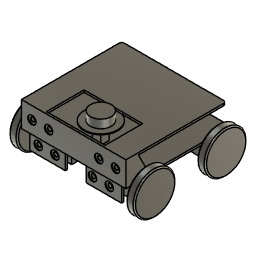
warehouse_robo v1 (Autodesk Fusion 360 design; units mm, degrees)
Autodesk Fusion 360 part; units mm, degrees
sketch "Sketch1" plane through (0, 0, 0) normal (0, 0, 1) x (1, 0, 0)
  line L0 (125, 125) -> (-125, 125)
  line L1 (-125, 125) -> (-125, -125)
  line L2 (-125, -125) -> (125, -125)
  line L3 (125, -125) -> (125, 125)
  line L4 (125, 125) -> (-125, -125) construction
  line L5 (-125, 125) -> (125, -125) construction
  dimension "d1" = 250
  dimension "d2" = 250
  constraint horizontal L0
  constraint perpendicular L0 L1
  constraint parallel L0 L2
  constraint parallel L1 L3
  constraint coincident L4 origin
  constraint coincident L5 origin
  measures "d1" distance of L1.end L2.end
  measures "d2" distance of L0.end L1.end
extrude "Extrude1" add sketch "Sketch1" along normal blind 5
sketch "Sketch2" plane through (0, 0, 0) normal (0, 1, 0) x (1, 0, 0)
  line L0 (-125, -5, -125) -> (-125, -55, -125)
  line L1 (-125, -55, -125) -> (125, -55, -125)
  line L2 (125, -55, -125) -> (125, -5, -125)
  line L3 (-125, -5, -125) -> (125, -5, -125)
  dimension "d5" = 50
  dimension "d6" = 250
  dimension "d7" = 250
extrude "Extrude2" add sketch "Sketch2" along normal blind 5 contours L0 L1 L2 L3 in plane through (0, -125, 0) normal (0, 1, 0)
sketch "Sketch3" plane through (125, 0, 0) normal (1, 0, 0) x (0, 1, 0)
  line L0 (-125, 0) -> (125, 0)
  line L1 (125, 0) -> (125, 5)
  line L2 (125, 5) -> (-120, 5)
  line L3 (-120, 5) -> (-120, 55)
  line L4 (-120, 55) -> (-125, 55)
  line L5 (-125, 55) -> (-125, 0)
  line L6 (-120, 5) -> (-120, 55)
  line L7 (-120, 55) -> (-95, 55)
  line L8 (-120, 5) -> (-70, 5)
  line L9 (-70, 5) -> (-95, 55)
  dimension "d10" = 25
  dimension "d11" = 50
  constraint coincident L2.end L3.start
  constraint coincident L3.end L4.start
  constraint perpendicular L3 L7
  constraint coincident L2 L8.end
  measures "d10" distance of L3.end L7.end
  measures "d11" distance of L2.end L8.end
sketch "Sketch4" plane through (-125, 0, 0) normal (-1, 0, 0) x (0, -1, 0)
  line L0 (-125, 0) -> (125, 0)
  line L1 (125, 0) -> (125, 55)
  line L2 (125, 55) -> (120, 55)
  line L3 (120, 55) -> (120, 5)
  line L4 (120, 5) -> (-125, 5)
  line L5 (-125, 5) -> (-125, 0)
  line L6 (120, 5) -> (120, 55)
  line L7 (120, 55) -> (95, 55)
  line L8 (120, 5) -> (70, 5)
  line L9 (95, 55) -> (70, 5)
  constraint coincident L3.end L4.start
  constraint coincident L2.end L3.start
  constraint perpendicular L3 L7
  constraint perpendicular L3 L8
extrude "Extrude3" add sketch "Sketch4" against normal blind 10 contours L3 L4 L6 L7 L8 L9
extrude "Extrude4" add sketch "Sketch3" against normal blind 10 contours L2 L3 L6 L7 L8 L9
sketch "Sketch5" plane through (0, 0, 55) normal (0, 0, 1) x (-1, 0, 0)
  line L0 (125, 125) -> (-125, 125)
  line L1 (-125, 125) -> (-125, 95)
  line L2 (-125, 95) -> (-115, 95)
  line L3 (-115, 95) -> (-115, 120)
  line L4 (-115, 120) -> (115, 120)
  line L5 (115, 120) -> (115, 95)
  line L6 (115, 95) -> (125, 95)
  line L7 (125, 95) -> (125, 125)
  line L8 (-125, 125) -> (-125, -115)
  line L9 (125, 125) -> (125, -115)
  line L10 (125, -115) -> (-125, -115)
  dimension "d18" = 240
  dimension "d19" = 240
  constraint coincident L0.end L1.start
  constraint perpendicular L2 L8
  constraint coincident L0.start L7.end
  constraint perpendicular L0 L9
  measures "d18" distance of L0.end L8.end
  measures "d19" distance of L0.start L9.end
sketch "Sketch6" plane through (0, 0, 55) normal (0, 0, 1) x (-1, 0, 0)
extrude "Extrude5" add sketch "Sketch5" along normal blind 5
sketch "Sketch7" plane through (0, -125, 0) normal (0, -1, 0) x (1, 0, 0)
  line L0 (-125, 0) -> (125, 0)
  line L1 (125, 0) -> (125, 60)
  line L2 (125, 60) -> (-125, 60)
  line L3 (-125, 60) -> (-125, 0)
  line L4 (125, 0) -> (125, 30)
  circle A0 centre (-100, 30) radius 10
  circle A1 centre (-60, 30) radius 10
  circle A2 centre (60, 30) radius 10
  circle A3 centre (100, 30) radius 10
  dimension "d22" = 20
  dimension "d23" = 20
  dimension "d24" = 20
  dimension "d25" = 20
  constraint coincident L0.end L1.start
  constraint midpoint L1 L4.end
  measures "d22" diameter of A0
  measures "d23" diameter of A1
  measures "d24" diameter of A2
  measures "d25" diameter of A3
extrude "Extrude6" cut sketch "Sketch7" against normal blind 2 contours A0 | A1 | A2 | A3
sketch "Sketch8" plane through (0, -123, 0) normal (0, -1, 0) x (1, 0, 0)
  circle A0 centre (-100, 30) radius 10
  circle A1 centre (-100, 30) radius 5
  dimension "d28" = 10
  constraint concentric A0 A1
  measures "d28" diameter of A1
sketch "Sketch9" plane through (0, -123, 0) normal (0, -1, 0) x (1, 0, 0)
  circle A0 centre (-60, 30) radius 10
  circle A1 centre (-60, 30) radius 5
  dimension "d29" = 10
  constraint concentric A0 A1
  measures "d29" diameter of A1
sketch "Sketch10" plane through (0, -123, 0) normal (0, -1, 0) x (1, 0, 0)
  circle A0 centre (60, 30) radius 10
  circle A1 centre (60, 30) radius 5
  dimension "d30" = 10
  constraint concentric A0 A1
  measures "d30" diameter of A1
sketch "Sketch11" plane through (0, -123, 0) normal (0, -1, 0) x (1, 0, 0)
  circle A0 centre (100, 30) radius 10
  circle A1 centre (100, 30) radius 5
  dimension "d31" = 10
  constraint concentric A0 A1
  measures "d31" diameter of A1
extrude "Extrude7" cut sketch "Sketch9" sketch "Sketch8" sketch "Sketch10" sketch "Sketch11" against normal blind 1 contours A1 of sketch 2 contours A1 of sketch 3 contours A1 of sketch 4 contours A1
sketch "Sketch12" plane through (0, 0, 60) normal (0, 0, 1) x (-1, 0, 0)
  line L0 (125, 125) -> (-125, 125)
  line L1 (-125, 125) -> (-125, -115)
  line L2 (-125, -115) -> (125, -115)
  line L3 (125, -115) -> (125, 125)
  line L4 (-125, 125) -> (-125, 120)
  line L5 (-125, 120) -> (125, 120)
  line L6 (125, 120) -> (70, 120)
  line L7 (70, 120) -> (70, 50)
  line L8 (-70, 120) -> (-70, 30)
  line L9 (-70, 30) -> (70, 30)
  line L10 (70, 30) -> (70, 50)
  dimension "d34" = 5
  constraint coincident L0.end L1.start
  constraint perpendicular L0 L4
  constraint coincident L3 L5.end
  constraint perpendicular L3 L5
  constraint coincident L5 L6.end
  constraint perpendicular L5 L7
  constraint coincident L5 L8.start
  constraint perpendicular L5 L8
  constraint perpendicular L1 L9
  constraint perpendicular L9 L10
  measures "d34" distance of L0.end L4.end
extrude "Extrude8" cut sketch "Sketch12" against normal blind 20 contours L5 L7 L8 L9 L10
sketch "Sketch13" plane through (0, 0, 5) normal (0, 0, 1) x (-1, 0, 0)
  line L0 (-115, 70) -> (-125, 70)
  line L1 (-125, 70) -> (-125, -125)
  line L2 (-125, -125) -> (125, -125)
  line L3 (125, -125) -> (125, 70)
  line L4 (125, 70) -> (115, 70)
  line L5 (115, 70) -> (115, 120)
  line L6 (115, 120) -> (-115, 120)
  line L7 (-115, 120) -> (-115, 70)
  line L8 (-10, 70) -> (10, 70)
  line L9 (10, 70) -> (10, 50)
  line L10 (10, 50) -> (-10, 50)
  line L11 (-10, 50) -> (-10, 70)
  line L12 (-10, 70) -> (10, 50) construction
  line L13 (10, 70) -> (-10, 50) construction
  point P0 (0, 60)
  constraint horizontal L8
  constraint perpendicular L8 L9
  constraint parallel L8 L10
  constraint parallel L9 L11
  constraint coincident L12 P0
  constraint coincident L13 P0
extrude "Extrude9" add sketch "Sketch13" along normal blind 40 contours L8 L9 L10 L11
sketch "Sketch14" plane through (0, 0, 45) normal (0, 0, 1) x (-1, 0, 0)
  line L0 (-10, 50) -> (10, 50)
  line L1 (10, 50) -> (10, 70)
  line L2 (10, 70) -> (-10, 70)
  line L3 (-10, 70) -> (-10, 50)
  circle A0 centre (0, 60) radius 40
extrude "Extrude10" add sketch "Sketch14" along normal blind 2 contours L0 L1 L2 L3 | A0
sketch "Sketch15" plane through (0, 0, 47) normal (0, 0, 1) x (-1, 0, 0)
  circle A0 centre (0, 60) radius 40
  circle A1 centre (0, 60) radius 25.0431
  constraint concentric A0 A1
extrude "Extrude11" add sketch "Sketch15" along normal blind 20 contours A1
sketch "Sketch16" plane through (0, 0, 0) normal (0, 0, -1) x (1, 0, 0)
  line L0 (125, -125) -> (125, 125)
  line L1 (125, 125) -> (-125, 125)
  line L2 (-125, 125) -> (-125, -125)
  line L3 (-125, -125) -> (125, -125)
  line L4 (-110, 120) -> (-25, 120)
  line L5 (-25, 120) -> (-25, 115)
  line L6 (-25, 115) -> (-110, 115)
  line L7 (-110, 115) -> (-110, 120)
  line L8 (110, 120) -> (25, 120)
  line L9 (25, 120) -> (25, 115)
  line L10 (25, 115) -> (110, 115)
  line L11 (110, 115) -> (110, 120)
  dimension "d43" = 85
  dimension "d44" = 5
  dimension "d45" = 85
  dimension "d46" = 5
  constraint horizontal L4
  constraint vertical L5
  constraint horizontal L6
  constraint vertical L7
  constraint horizontal L8
  constraint vertical L9
  constraint horizontal L10
  constraint vertical L11
  measures "d43" distance of L4.start L4.end
  measures "d44" distance of L4.start L6.end
  measures "d45" distance of L8.start L8.end
  measures "d46" distance of L8.start L10.end
extrude "Extrude12" add sketch "Sketch16" along normal blind 40 contours L4 L5 L6 L7 | L8 L9 L10 L11
sketch "Sketch17" plane through (0, -120, 0) normal (0, -1, 0) x (1, 0, 0)
  line L0 (-25, 0) -> (-110, 0)
  line L1 (-110, 0) -> (-110, -40)
  line L2 (-110, -40) -> (-25, -40)
  line L3 (-25, -40) -> (-25, 0)
  circle A0 centre (-90, -20) radius 10
  circle A1 centre (-50, -20) radius 10
  circle A2 centre (40, -20) radius 10
  circle A3 centre (80, -20) radius 10
  dimension "d49" = 20
  dimension "d50" = 20
  dimension "d51" = 20
  dimension "d52" = 20
  measures "d49" diameter of A0
  measures "d50" diameter of A1
  measures "d51" diameter of A2
  measures "d52" diameter of A3
extrude "Extrude13" cut sketch "Sketch17" against normal blind 2 contours A0 | A1 | A2 | A3
sketch "Sketch18" plane through (0, -118, 0) normal (0, -1, 0) x (1, 0, 0)
  circle A0 centre (-90, -20) radius 10
  circle A1 centre (-90, -20) radius 5
  dimension "d55" = 10
  constraint concentric A0 A1
  measures "d55" diameter of A1
sketch "Sketch19" plane through (0, -118, 0) normal (0, -1, 0) x (1, 0, 0)
  circle A0 centre (-50, -20) radius 10
  circle A1 centre (-50, -20) radius 5
  dimension "d56" = 10
  constraint concentric A0 A1
  measures "d56" diameter of A1
sketch "Sketch20" plane through (0, -118, 0) normal (0, -1, 0) x (1, 0, 0)
  circle A0 centre (40, -20) radius 10
  circle A1 centre (40, -20) radius 5
  dimension "d57" = 10
  constraint concentric A0 A1
  measures "d57" diameter of A1
sketch "Sketch21" plane through (0, -118, 0) normal (0, -1, 0) x (1, 0, 0)
  circle A0 centre (80, -20) radius 10
  circle A1 centre (80, -20) radius 5
  dimension "d58" = 10
  constraint concentric A0 A1
  measures "d58" diameter of A1
extrude "Extrude14" cut sketch "Sketch20" sketch "Sketch21" sketch "Sketch19" sketch "Sketch18" against normal blind 1 contours A1 of sketch 2 contours A1 of sketch 3 contours A1 of sketch 4 contours A1
sketch "Sketch22" plane through (0, 0, 0) normal (0, 0, -1) x (1, 0, 0)
  line L0 (110, 115) -> (25, 115)
  line L1 (25, 115) -> (25, 120)
  line L2 (25, 120) -> (110, 120)
  line L3 (110, 120) -> (110, 115)
  line L4 (-110, 115) -> (-110, 120)
  line L5 (-110, 120) -> (-25, 120)
  line L6 (-25, 120) -> (-25, 115)
  line L7 (-25, 115) -> (-110, 115)
  line L8 (125, -125) -> (125, 125)
  line L9 (125, 125) -> (-125, 125)
  line L10 (-125, 125) -> (-125, -125)
  line L11 (-125, -125) -> (125, -125)
  line L12 (-110, 100) -> (-30, 100)
  line L13 (-30, 100) -> (-30, 60)
  line L14 (-30, 60) -> (-110, 60)
  line L15 (-110, 60) -> (-110, 100)
  line L16 (110, 100) -> (30, 100)
  line L17 (30, 100) -> (30, 60)
  line L18 (30, 60) -> (110, 60)
  line L19 (110, 60) -> (110, 100)
  line L20 (-110, -110) -> (-30, -110)
  line L21 (-30, -110) -> (-30, -70)
  line L22 (-30, -70) -> (-110, -70)
  line L23 (-110, -70) -> (-110, -110)
  line L24 (110, -110) -> (30, -110)
  line L25 (30, -110) -> (30, -70)
  line L26 (30, -70) -> (110, -70)
  line L27 (110, -70) -> (110, -110)
  dimension "d61" = 80
  dimension "d62" = 40
  constraint horizontal L12
  constraint vertical L13
  constraint horizontal L14
  constraint vertical L15
  constraint horizontal L16
  constraint vertical L17
  constraint horizontal L18
  constraint vertical L19
  constraint horizontal L20
  constraint vertical L21
  constraint horizontal L22
  constraint vertical L23
  constraint horizontal L24
  constraint vertical L25
  constraint horizontal L26
  constraint vertical L27
  measures "d61" distance of L24.start L24.end
  measures "d62" distance of L24.start L26.end
extrude "Extrude15" add sketch "Sketch22" along normal blind 40 contours L12 L13 L14 L15 | L16 L17 L18 L19 | L20 L21 L22 L23 | L24 L25 L26 L27
sketch "Sketch23" plane through (110, 0, 0) normal (1, 0, 0) x (0, 1, 0)
  line L0 (-60, 0) -> (-100, 0)
  line L1 (-100, 0) -> (-100, -40)
  line L2 (-100, -40) -> (-60, -40)
  line L3 (-60, -40) -> (-60, 0)
  circle A0 centre (-80, -20) radius 5
  dimension "d65" = 10
  measures "d65" diameter of A0
sketch "Sketch24" plane through (110, 0, 0) normal (1, 0, 0) x (0, 1, 0)
  line L0 (110, 0) -> (70, 0)
  line L1 (70, 0) -> (70, -40)
  line L2 (70, -40) -> (110, -40)
  line L3 (110, -40) -> (110, 0)
  circle A0 centre (90, -20) radius 5
  dimension "d66" = 10
  measures "d66" diameter of A0
sketch "Sketch25" plane through (-110, 0, 0) normal (-1, 0, 0) x (0, -1, 0)
  line L0 (-70, 0) -> (-110, 0)
  line L1 (-110, 0) -> (-110, -40)
  line L2 (-110, -40) -> (-70, -40)
  line L3 (-70, -40) -> (-70, 0)
  circle A0 centre (-90, -20) radius 5
  dimension "d67" = 10
  measures "d67" diameter of A0
sketch "Sketch26" plane through (-110, 0, 0) normal (-1, 0, 0) x (0, -1, 0)
  line L0 (100, 0) -> (60, 0)
  line L1 (60, 0) -> (60, -40)
  line L2 (60, -40) -> (100, -40)
  line L3 (100, -40) -> (100, 0)
  circle A0 centre (80, -20) radius 5
  dimension "d68" = 10
  measures "d68" diameter of A0
extrude "Extrude16" add sketch "Sketch26" sketch "Sketch25" along normal blind 20 contours A0 of sketch 2 contours A0
extrude "Extrude17" add sketch "Sketch23" sketch "Sketch24" along normal blind 20 contours A0 of sketch 2 contours A0
sketch "Sketch27" plane through (130, 0, 0) normal (1, 0, 0) x (0, 1, 0)
  circle A0 centre (-80, -20) radius 5
  circle A1 centre (-80, -20) radius 50
  dimension "d73" = 100
  constraint concentric A0 A1
  measures "d73" diameter of A1
sketch "Sketch28" plane through (130, 0, 0) normal (1, 0, 0) x (0, 1, 0)
  circle A0 centre (90, -20) radius 5
  circle A1 centre (90, -20) radius 50
  dimension "d74" = 100
  constraint concentric A0 A1
  measures "d74" diameter of A1
sketch "Sketch29" plane through (-130, 0, 0) normal (-1, 0, 0) x (0, -1, 0)
  circle A0 centre (80, -20) radius 5
  circle A1 centre (80, -20) radius 50
  dimension "d75" = 100
  constraint concentric A0 A1
  measures "d75" diameter of A1
sketch "Sketch30" plane through (-130, 0, 0) normal (-1, 0, 0) x (0, -1, 0)
  circle A0 centre (-90, -20) radius 5
  circle A1 centre (-90, -20) radius 50
  dimension "d76" = 100
  constraint concentric A0 A1
  measures "d76" diameter of A1
extrude "Extrude18" add sketch "Sketch28" sketch "Sketch27" along normal blind 20 contours A0 | A1 of sketch 2 contours A0 | A1
extrude "Extrude19" add sketch "Sketch29" sketch "Sketch30" along normal blind 20 contours A0 | A1 of sketch 2 contours A0 | A1
fillet "Fillet1" radius 3 2 edges at (150, -126.6164, -38.0808) (130, -126.6164, -38.0808)
fillet "Fillet2" radius 3 2 edges at (150, 43.3836, -38.0808) (130, 43.3836, -38.0808)
fillet "Fillet3" radius 3 2 edges at (-130, -33.3836, -38.0808) (-150, -33.3836, -38.0808)
fillet "Fillet4" radius 3 2 edges at (-150, 136.6164, -38.0808) (-130, 136.6164, -38.0808)
fillet "Fillet5" radius 6 2 edges at (125, 115, 57.5) (-125, 115, 57.5)
